Autodesk Fusion 360 part; units mm, degrees
note: some values were not read from the file. Chosen so that the rebuilt part matches the saved one: which face or edge a step refers to; which pieces of a blend or face edit are solid. Set by a fixed rule: which sketch regions a step uses.
(part 5 of 5)
extrude "押し出し16" cut sketch "スケッチ7" against normal blind 100 contours A83 A84 L25 A370 L551 L560 A378 A381 A386 A401 L597 | L24 A72 A73 A203 A210 A215 L242 L243 L244 A223 A235 | L27 A87 A88 A178 A187 A202 A206 L641 L644 A435 A436 L651 L655 L658 A438 A439 A440 | A68 A69 L22 A179 A185 L252 L253 L255 A221 A222 A231 | A66 A67 A68 L33 A99 L66 L67 A157 L68 A159 L70 L71 A162 A179 A185 | L30 A94 A95 L131 L165 A239 A240 A243 A247 L337 L411 A308 A317 A324 A332 A361 L614 | A95 A96 L31 L90 L139 A363 A367 L540 A372 A375 A377 bodies 1
extrude "押し出し17" cut sketch "スケッチ7" against normal blind 100 contours A88 A89 A90 A91 L28 A178 A187 A202 A206 L415 L417 L419 L423 L434 L443 L444 A341 A344 A345 L470 A346 A355 L503 bodies 1
extrude "押し出し5" [suppressed]
extrude "押し出し6" [suppressed]
extrude "押し出し7" [suppressed]
sketch "スケッチ3" plane through (0, 0, 1.5) normal (0, 0, 1) x (-1, 0, 0)
  arc A0 (-33.7586, -84.6686) -> (-33.8139, -77.6537) centre (-37.3495, -81.1892) ccw
  line L0 (-33.8139, -77.6537) -> (-38.5865, -72.8811)
  arc A1 (-38.9491, -66.2144) -> (-38.5865, -72.8811) centre (-35.0509, -69.3456) ccw
  arc A2 (-38.9441, -66.1678) -> (-38.9491, -66.2144) centre (-33.9744, -66.7173) ccw
  line L1 (-38.9441, -66.1678) -> (-15.8059, -43.0296)
  arc A3 (-10.9963, -41.7301) -> (-15.8059, -43.0296) centre (-12.2704, -46.5651) ccw
  arc A4 (-10.9963, -41.7301) -> (10.9963, -41.7301) centre (0, 0) ccw
  arc A5 (15.8059, -43.0296) -> (10.9963, -41.7301) centre (12.2704, -46.5651) ccw
  line L2 (15.8059, -43.0296) -> (38.9441, -66.1678)
  arc A6 (38.6046, -72.863) -> (38.9441, -66.1678) centre (35.0691, -69.3275) ccw
  line L3 (38.6046, -72.863) -> (33.8135, -77.6541)
  arc A7 (33.8135, -77.6541) -> (33.7038, -84.612) centre (37.349, -81.1896) ccw
  line L4 (33.7038, -84.612) -> (33.8135, -84.7252)
  line L5 (33.8135, -84.7252) -> (37.0951, -88.0068)
  arc A8 (35.2806, -96.2368) -> (37.0951, -88.0068) centre (33.5596, -91.5424) ccw
  arc A9 (-35.2806, -96.2368) -> (35.2806, -96.2368) centre (0, 0) ccw
  arc A10 (-37.0951, -88.0068) -> (-35.2806, -96.2368) centre (-33.5596, -91.5424) ccw
  line L6 (-37.0951, -88.0068) -> (-33.8135, -84.7252)
  line L7 (-33.8135, -84.7252) -> (-33.7586, -84.6686)
  arc A11 (-62.6322, -42.4797) -> (-62.2927, -49.1749) centre (-58.7571, -45.6394) ccw
  line L8 (-62.6322, -42.4797) -> (-43.4926, -23.3401)
  arc A12 (-35.8083, -24.0851) -> (-43.4926, -23.3401) centre (-39.9571, -26.8756) ccw
  arc A13 (-35.8083, -24.0851) -> (-24.0851, -35.8083) centre (0, 0) ccw
  arc A14 (-23.3401, -43.4926) -> (-24.0851, -35.8083) centre (-26.8756, -39.9571) ccw
  line L9 (-23.3401, -43.4926) -> (-42.122, -62.2745)
  arc A15 (-49.1931, -62.2745) -> (-42.122, -62.2745) centre (-45.6575, -58.739) ccw
  line L10 (-49.1931, -62.2745) -> (-62.2927, -49.1749)
  arc A16 (42.4797, -62.6322) -> (49.1749, -62.2927) centre (45.6394, -58.7571) ccw
  line L11 (42.4797, -62.6322) -> (23.3401, -43.4926)
  arc A17 (24.0851, -35.8083) -> (23.3401, -43.4926) centre (26.8756, -39.9571) ccw
  arc A18 (24.0851, -35.8083) -> (35.8083, -24.0851) centre (0, 0) ccw
  arc A19 (43.4926, -23.3401) -> (35.8083, -24.0851) centre (39.9571, -26.8756) ccw
  line L12 (43.4926, -23.3401) -> (62.2745, -42.122)
  arc A20 (62.2745, -49.1931) -> (62.2745, -42.122) centre (58.739, -45.6575) ccw
  line L13 (62.2745, -49.1931) -> (49.1749, -62.2927)
  line L14 (65.8101, -38.5865) -> (63.9577, -36.7341)
  line L15 (63.9577, -36.7341) -> (43.0296, -15.8059)
  arc A21 (41.7301, -10.9963) -> (43.0296, -15.8059) centre (46.5651, -12.2704) ccw
  arc A22 (41.7301, -10.9963) -> (41.7301, 10.9963) centre (0, 0) ccw
  arc A23 (43.0296, 15.8059) -> (41.7301, 10.9963) centre (46.5651, 12.2704) ccw
  line L16 (43.0296, 15.8059) -> (66.1678, 38.9441)
  arc A24 (72.863, 38.6046) -> (66.1678, 38.9441) centre (69.3275, 35.0691) ccw
  line L17 (72.863, 38.6046) -> (77.6541, 33.8135)
  arc A25 (77.6541, 33.8135) -> (84.7252, 33.8135) centre (81.1896, 37.349) ccw
  line L18 (84.7252, 33.8135) -> (88.0068, 37.0951)
  arc A26 (96.2368, 35.2806) -> (88.0068, 37.0951) centre (91.5424, 33.5596) ccw
  arc A27 (96.2368, -35.2806) -> (96.2368, 35.2806) centre (0, 0) ccw
  arc A28 (88.0068, -37.0951) -> (96.2368, -35.2806) centre (91.5424, -33.5596) ccw
  line L19 (88.0068, -37.0951) -> (84.7252, -33.8135)
  arc A29 (84.7252, -33.8135) -> (77.6541, -33.8135) centre (81.1896, -37.349) ccw
  line L20 (77.6541, -33.8135) -> (72.8811, -38.5865)
  arc A30 (65.8101, -38.5865) -> (72.8811, -38.5865) centre (69.3456, -35.0509) ccw
  circle A31 centre (26.1275, 49.8155) radius 1.75
  circle A32 centre (39.2089, 15.5208) radius 1.75
  circle A33 centre (15.5208, 39.2089) radius 1.75
  circle A34 centre (49.8155, 26.1275) radius 1.75
  arc A35 (91.4938, -47.061) -> (90.783, -46.7156) centre (91.0045, -47.1639) ccw
  arc A36 (91.4938, -47.061) -> (97.869, -44.4738) centre (93.3169, -42.4052) ccw
  arc A37 (97.869, -44.4738) -> (97.869, 44.4738) centre (0, 0) ccw
  arc A38 (97.869, 44.4738) -> (89.7814, 45.9408) centre (93.3169, 42.4052) ccw
  line L21 (89.7814, 45.9408) -> (84.7252, 40.8846)
  arc A39 (77.6541, 40.8846) -> (84.7252, 40.8846) centre (81.1896, 44.4201) ccw
  line L22 (77.6541, 40.8846) -> (40.8846, 77.6541)
  arc A40 (40.8846, 84.7252) -> (40.8846, 77.6541) centre (44.4201, 81.1896) ccw
  line L23 (40.8846, 84.7252) -> (45.9408, 89.7814)
  arc A41 (45.9408, 89.7814) -> (44.4738, 97.869) centre (42.4052, 93.3169) ccw
  arc A42 (44.4738, 97.869) -> (37.9262, 100.5876) centre (0, 0) ccw
  arc A43 (37.9256, 100.5859) -> (37.9262, 100.5876) centre (0, 113.3) ccw
  arc A44 (37.9256, 100.5859) -> (37.8014, 100.6345) centre (36.0432, 95.9538) ccw
  arc A45 (37.8014, 100.6345) -> (29.5575, 103.3567) centre (0, 0) ccw
  arc A46 (29.5575, 103.3567) -> (23.7528, 100.868) centre (28.1827, 98.5494) ccw
  arc A47 (-23.7528, 100.868) -> (23.7528, 100.868) centre (0, 113.3) ccw
  arc A48 (-23.7528, 100.868) -> (-29.5575, 103.3567) centre (-28.1827, 98.5494) ccw
  arc A49 (-29.5575, 103.3567) -> (-37.8014, 100.6345) centre (0, 0) ccw
  arc A50 (-37.8014, 100.6345) -> (-37.9256, 100.5859) centre (-36.0432, 95.9538) ccw
  arc A51 (-37.9262, 100.5876) -> (-37.9256, 100.5859) centre (0, 113.3) ccw
  arc A52 (-37.9262, 100.5876) -> (-44.4738, 97.869) centre (0, 0) ccw
  arc A53 (-44.4738, 97.869) -> (-45.9408, 89.7814) centre (-42.4052, 93.3169) ccw
  line L24 (-45.9408, 89.7814) -> (-40.8846, 84.7252)
  arc A54 (-40.8846, 77.6541) -> (-40.8846, 84.7252) centre (-44.4201, 81.1896) ccw
  line L25 (-40.8846, 77.6541) -> (-77.6541, 40.8846)
  arc A55 (-84.7252, 40.8846) -> (-77.6541, 40.8846) centre (-81.1896, 44.4201) ccw
  line L26 (-84.7252, 40.8846) -> (-89.7814, 45.9408)
  arc A56 (-89.7814, 45.9408) -> (-97.869, 44.4738) centre (-93.3169, 42.4052) ccw
  arc A57 (-97.869, 44.4738) -> (-97.869, -44.4738) centre (0, 0) ccw
  arc A58 (-97.869, -44.4738) -> (-91.4938, -47.061) centre (-93.3169, -42.4052) ccw
  arc A59 (-90.783, -46.7156) -> (-91.4938, -47.061) centre (-91.0045, -47.1639) ccw
  arc A60 (-90.783, -46.7156) -> (-89.7814, -45.9408) centre (-93.3169, -42.4052) ccw
  line L27 (-89.7814, -45.9408) -> (-84.7252, -40.8846)
  arc A61 (-77.6541, -40.8846) -> (-84.7252, -40.8846) centre (-81.1896, -44.4201) ccw
  line L28 (-77.6541, -40.8846) -> (-40.8846, -77.6541)
  arc A62 (-40.8846, -84.7252) -> (-40.8846, -77.6541) centre (-44.4201, -81.1896) ccw
  line L29 (-40.8846, -84.7252) -> (-45.9408, -89.7814)
  arc A63 (-45.9408, -89.7814) -> (-44.4738, -97.869) centre (-42.4052, -93.3169) ccw
  arc A64 (-44.4738, -97.869) -> (44.4738, -97.869) centre (0, 0) ccw
  arc A65 (44.4738, -97.869) -> (45.9408, -89.7814) centre (42.4052, -93.3169) ccw
  line L30 (45.9408, -89.7814) -> (40.8846, -84.7252)
  arc A66 (40.8846, -77.6541) -> (40.8846, -84.7252) centre (44.4201, -81.1896) ccw
  line L31 (40.8846, -77.6541) -> (77.6541, -40.8846)
  arc A67 (84.7252, -40.8846) -> (77.6541, -40.8846) centre (81.1896, -44.4201) ccw
  line L32 (84.7252, -40.8846) -> (89.7814, -45.9408)
  arc A68 (89.7814, -45.9408) -> (90.783, -46.7156) centre (93.3169, -42.4052) ccw
  line L33 (-63.9577, -36.7341) -> (-66.1678, -38.9441)
  arc A69 (-72.863, -38.6046) -> (-66.1678, -38.9441) centre (-69.3275, -35.0691) ccw
  line L34 (-72.863, -38.6046) -> (-77.6541, -33.8135)
  arc A70 (-77.6541, -33.8135) -> (-84.7252, -33.8135) centre (-81.1896, -37.349) ccw
  line L35 (-84.7252, -33.8135) -> (-88.0068, -37.0951)
  arc A71 (-96.2368, -35.2806) -> (-88.0068, -37.0951) centre (-91.5424, -33.5596) ccw
  arc A72 (-96.2368, 35.2806) -> (-96.2368, -35.2806) centre (0, 0) ccw
  arc A73 (-88.0068, 37.0951) -> (-96.2368, 35.2806) centre (-91.5424, 33.5596) ccw
  line L36 (-88.0068, 37.0951) -> (-84.7252, 33.8135)
  arc A74 (-84.7252, 33.8135) -> (-77.6541, 33.8135) centre (-81.1896, 37.349) ccw
  line L37 (-77.6541, 33.8135) -> (-72.863, 38.6046)
  arc A75 (-66.1678, 38.9441) -> (-72.863, 38.6046) centre (-69.3275, 35.0691) ccw
  line L38 (-66.1678, 38.9441) -> (-43.0296, 15.8059)
  arc A76 (-41.7301, 10.9963) -> (-43.0296, 15.8059) centre (-46.5651, 12.2704) ccw
  arc A77 (-41.7301, 10.9963) -> (-41.7301, -10.9963) centre (0, 0) ccw
  arc A78 (-43.0296, -15.8059) -> (-41.7301, -10.9963) centre (-46.5651, -12.2704) ccw
  line L39 (-43.0296, -15.8059) -> (-63.9577, -36.7341)
  line L40 (62.6322, 42.4797) -> (43.4926, 23.3401)
  arc A79 (35.8083, 24.0851) -> (43.4926, 23.3401) centre (39.9571, 26.8756) ccw
  arc A80 (35.8083, 24.0851) -> (24.0851, 35.8083) centre (0, 0) ccw
  arc A81 (23.3401, 43.4926) -> (24.0851, 35.8083) centre (26.8756, 39.9571) ccw
  line L41 (23.3401, 43.4926) -> (42.122, 62.2745)
  arc A82 (49.1931, 62.2745) -> (42.122, 62.2745) centre (45.6575, 58.739) ccw
  line L42 (49.1931, 62.2745) -> (62.2927, 49.1749)
  arc A83 (62.6322, 42.4797) -> (62.2927, 49.1749) centre (58.7571, 45.6394) ccw
  line L43 (38.5865, 65.8101) -> (15.8059, 43.0296)
  arc A84 (10.9963, 41.7301) -> (15.8059, 43.0296) centre (12.2704, 46.5651) ccw
  arc A85 (10.9963, 41.7301) -> (-10.9963, 41.7301) centre (0, 0) ccw
  arc A86 (-15.8059, 43.0296) -> (-10.9963, 41.7301) centre (-12.2704, 46.5651) ccw
  line L44 (-15.8059, 43.0296) -> (-38.5865, 65.8101)
  arc A87 (-38.5865, 72.8811) -> (-38.5865, 65.8101) centre (-35.0509, 69.3456) ccw
  line L45 (-38.5865, 72.8811) -> (-24.7285, 86.7391)
  arc A88 (-18.3143, 87.2917) -> (-24.7285, 86.7391) centre (-21.193, 83.2035) ccw
  arc A89 (-18.3143, 87.2917) -> (18.3143, 87.2917) centre (0, 113.3) ccw
  arc A90 (24.7285, 86.7391) -> (18.3143, 87.2917) centre (21.193, 83.2035) ccw
  line L46 (24.7285, 86.7391) -> (38.5865, 72.8811)
  arc A91 (38.5865, 65.8101) -> (38.5865, 72.8811) centre (35.0509, 69.3456) ccw
  arc A92 (17.125, 34.0956) -> (-17.125, 34.0956) centre (0, 0) ccw
  line L47 (17.125, 34.0956) -> (17.1965, 34.167)
  line L48 (17.1965, 34.167) -> (17.4152, 33.9483)
  arc A93 (33.9483, 17.4152) -> (17.4152, 33.9483) centre (0, 0) ccw
  line L49 (33.9483, 17.4152) -> (34.167, 17.1965)
  line L50 (34.167, 17.1965) -> (34.0956, 17.125)
  arc A94 (-34.0956, 17.125) -> (34.0956, 17.125) centre (0, 0) ccw
  line L51 (-34.0956, 17.125) -> (-34.167, 17.1965)
  line L52 (-34.167, 17.1965) -> (-33.9483, 17.4152)
  arc A95 (-17.4152, 33.9483) -> (-33.9483, 17.4152) centre (0, 0) ccw
  line L53 (-17.4152, 33.9483) -> (-17.1965, 34.167)
  line L54 (-17.1965, 34.167) -> (-17.125, 34.0956)
  line L55 (40.3326, 91.2443) -> (35.2277, 86.1394)
  arc A96 (32.3993, 86.1394) -> (35.2277, 86.1394) centre (33.8135, 87.5536) ccw
  line L56 (32.3993, 86.1394) -> (26.1835, 92.3551)
  arc A97 (25.9652, 94.9247) -> (26.1835, 92.3551) centre (27.5978, 93.7693) ccw
  arc A98 (25.9652, 94.9247) -> (26.3162, 95.431) centre (0, 113.3) ccw
  arc A99 (32.0144, 97.3721) -> (26.3162, 95.431) centre (30.4528, 92.6222) ccw
  arc A100 (39.6929, 94.5025) -> (32.0144, 97.3721) centre (0, 0) ccw
  arc A101 (40.3326, 91.2443) -> (39.6929, 94.5025) centre (38.9184, 92.6585) ccw
  circle A102 centre (-39.2089, -15.5208) radius 1.75
  circle A103 centre (-15.5208, -39.2089) radius 1.75
  circle A104 centre (-39.2089, 15.5208) radius 1.75
  circle A105 centre (-26.1275, -49.8155) radius 1.75
  circle A106 centre (-15.5208, 39.2089) radius 1.75
  circle A107 centre (-49.8155, 26.1275) radius 1.75
  circle A108 centre (-49.8155, -26.1275) radius 1.75
  arc A109 (-24.0851, 35.8083) -> (-23.3401, 43.4926) centre (-26.8756, 39.9571) ccw
  arc A110 (-24.0851, 35.8083) -> (-35.8083, 24.0851) centre (0, 0) ccw
  arc A111 (-43.4926, 23.3401) -> (-35.8083, 24.0851) centre (-39.9571, 26.8756) ccw
  line L57 (-43.4926, 23.3401) -> (-62.6322, 42.4797)
  arc A112 (-62.2927, 49.1749) -> (-62.6322, 42.4797) centre (-58.7571, 45.6394) ccw
  line L58 (-62.2927, 49.1749) -> (-49.1931, 62.2745)
  arc A113 (-42.122, 62.2745) -> (-49.1931, 62.2745) centre (-45.6575, 58.739) ccw
  line L59 (-42.122, 62.2745) -> (-23.3401, 43.4926)
  circle A114 centre (-26.1275, 49.8155) radius 1.75
  arc A115 (-35.2277, 86.1394) -> (-32.3993, 86.1394) centre (-33.8135, 87.5536) ccw
  line L60 (-35.2277, 86.1394) -> (-40.3326, 91.2443)
  arc A116 (-39.6929, 94.5025) -> (-40.3326, 91.2443) centre (-38.9184, 92.6585) ccw
  arc A117 (-32.0144, 97.3721) -> (-39.6929, 94.5025) centre (0, 0) ccw
  arc A118 (-26.3162, 95.431) -> (-32.0144, 97.3721) centre (-30.4528, 92.6222) ccw
  arc A119 (-26.3162, 95.431) -> (-25.9652, 94.9247) centre (0, 113.3) ccw
  arc A120 (-26.1835, 92.3551) -> (-25.9652, 94.9247) centre (-27.5978, 93.7693) ccw
  line L61 (-26.1835, 92.3551) -> (-32.3993, 86.1394)
  circle A121 centre (49.8155, -26.1275) radius 1.75
  circle A122 centre (26.1275, -49.8155) radius 1.75
  circle A123 centre (15.5208, -39.2089) radius 1.75
  circle A124 centre (39.2089, -15.5208) radius 1.75
  circle A125 centre (32.1379, -59.3615) radius 5
  circle A126 centre (32.1379, -59.3615) radius 1.75
  circle A127 centre (-32.1379, -59.3615) radius 1.75
  circle A128 centre (-32.1379, -59.3615) radius 5
  circle A129 centre (32.1379, -59.3615) radius 2.5
  circle A130 centre (-32.1379, -59.3615) radius 2.5
  dimension "d72" = 3.5
  dimension "d73" = 3.5
  dimension "d74" = 5
  dimension "d75" = 5
  constraint concentric A127 A128
  constraint concentric A125 A129
  constraint concentric A128 A130
  measures "d72" diameter of A126
  measures "d73" diameter of A127
  measures "d74" diameter of A129
  measures "d75" diameter of A130
extrude "押し出し8" [suppressed]
extrude "押し出し9" [suppressed]
fillet "フィレット3" [suppressed]
